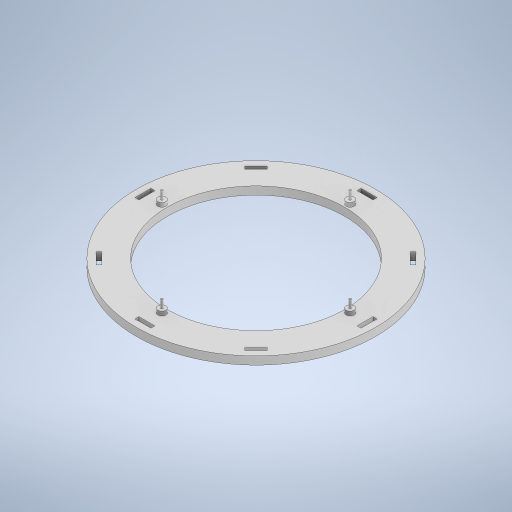
# Autodesk Inventor part: TableCover
Saved by Autodesk Inventor 2023 (Build 270158000, 158)
## iProperties
Created: 2023-03-23
Part Number: TableCover
Material: Generic
Document SubType Name: Modeling
Designer: czapa
Density: 1 g/cm^3
Appearance: Default
Author: czapa
Autodesk Inventor part; units mm, degrees
ref_plane "YZ Plane" through (0, 0, 0) normal (1, 0, 0) x (0, 1, 0)
ref_plane "XZ Plane" through (0, 0, 0) normal (0, 1, 0) x (-1, 0, 0)
ref_plane "XY Plane" through (0, 0, 0) normal (0, 0, 1) x (1, 0, 0)
sketch "Sketch2" plane through (0, 0, 0) normal (0, 1, 0) x (-1, 0, 0)
  circle A0 centre (0, 0) radius 150
  dimension "d1" = 300
  constraints: 1 centre point, 1 coincident
  measures "d1" diameter of A0
extrude "Extrusion1" add sketch "Sketch2" along normal blind 10
sketch "Sketch3" plane through (0, 10, 0) normal (0, 1, 0) x (1, 0, 0)
  circle A0 centre (0, 0) radius 111.25
  dimension "d4" = 222.5
  constraints: 1 centre point, 1 coincident
  measures "d4" diameter of A0
sketch "Sketch4" plane through (0, 10, 0) normal (0, 1, 0) x (1, 0, 0)
  circle A0 centre (0, 0) radius 118.125
  circle A1 centre (0, 118.125) radius 1.25
  dimension "d5" = 236.25
  dimension "d6" = 2.5
  constraints: 2 coincident, 1 centre point, 1 vertical alignment, 2 other
  measures "d6" diameter of A1
extrude "Extrusion2" add sketch "Sketch4" along normal blind 15 contours A1 A0 | A0 A1 picked at (0.0501, 117.7109) picked at (0.0492, 118.5383)
sketch "Sketch5" plane through (0, 10, 0) normal (0, 1, 0) x (1, 0, 0)
  circle A0 centre (0, 118.125) radius 1.25 projected
  circle A1 centre (0, 118.125) radius 5
  point P0 (0, 0)
  dimension "d9" = 10
  constraints: 1 centre point, 1 coincident
  measures "d9" diameter of A1
extrude "Extrusion3" add sketch "Sketch5" along normal blind 5
extrude "Extrusion4" cut sketch "Sketch3" against normal blind 10
pattern_circular "Circular Pattern1" count 4 over 360 about axis through (0, -10, 0) along (0, 1, 0) of "Extrusion3", "Extrusion2"
sketch "Sketch6" plane through (0, 10, 0) normal (0, 1, 0) x (1, 0, 0)
  line L0 (0, -139.3513) -> (10, -139.3513)
  line L1 (0, -139.3513) -> (10, -139.3513) construction
  line L2 (10, -139.3513) -> (10, -141.8513)
  line L3 (10, -141.8513) -> (-10, -141.8513)
  line L4 (-10, -141.8513) -> (-10, -136.8513)
  line L5 (-10, -136.8513) -> (10, -136.8513)
  line L6 (10, -136.8513) -> (10, -141.8513)
  point P0 (0, 0)
  dimension "d17" = 10
  dimension "d18" = 0
  dimension "d19" = 2.5
  dimension "d20" = 20
  dimension "d21" = 5
  constraints: 14 end point, 3 horizontal, 2 parallel, 2 perpendicular, 1 collinear
  measures "d17" distance of L0.start L0.end
  measures "d18" distance between parallel lines of L0 L1
  measures "d19" distance of L0.end L2.end
  measures "d20" distance of L4.end L5.end
  measures "d21" distance of L3.end L4.end
extrude "Extrusion5" cut sketch "Sketch6" against normal up to surface (10 mm away)
pattern_circular "Circular Pattern2" count 8 over 360 about axis through (0, -10, 0) along (0, 1, 0) of "Extrusion5"
body "Solid1"
